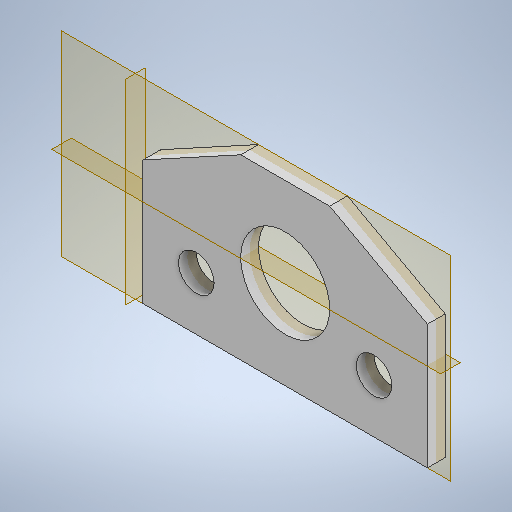
# Autodesk Inventor part: chap2ex3
Saved by Autodesk Inventor 2025.2 (Build 292293000, 293)
## iProperties
Created: 2025-01-31
Part Number: chap2ex3
Material: Generic
Document SubType Name: Modeling
Designer: Moofin
Density: 1 g/cm^3
Appearance: Default
Author: Moofin
Autodesk Inventor part; units mm, degrees
sketch "Sketch1" plane through (0, 0, 0) normal (0, 0, 1) x (1, 0, 0)
  line L0 (5.8796, 31.75) -> (107.4796, 31.75)
  line L1 (107.4796, 31.75) -> (107.4796, -31.75)
  line L2 (107.4796, -31.75) -> (5.8796, -31.75)
  line L3 (5.8796, -31.75) -> (5.8796, 31.75)
  line L4 (-21.4959, 0) -> (128.9756, 0) projected
  point P0 (0, 0)
  dimension "d0" = 63.5
  dimension "d1" = 101.6
  dimension "d2" = 31.75
  constraints: 8 end point, 2 parallel, 1 horizontal, 1 perpendicular
  measures "d0" distance between parallel lines of L2 L0
  measures "d1" distance between parallel lines of L1 L3
  measures "d2" distance between parallel lines of L4 L0
extrude "Extrusion1" add sketch "Sketch1" along normal mid plane 6.35
sketch "Sketch2" plane through (0, 0, 3.175) normal (0, 0, 1) x (1, 0, 0)
  circle A0 centre (56.6796, 0) radius 15.875
  circle A1 centre (24.9296, -12.7) radius 6.35
  line L0 (5.8796, -31.75) -> (107.4796, -31.75) projected
  line L1 (5.8796, 31.75) -> (5.8796, -31.75) projected
  circle A2 centre (88.4296, -12.7) radius 6.35
  line L2 (107.4796, -31.75) -> (107.4796, 31.75) projected
  line L3 (107.4796, 31.75) -> (5.8796, 31.75) projected
  point P0 (0, 0)
  dimension "d5" = 31.75
  dimension "d6" = 12.7
  dimension "d8" = 19.05
  dimension "d9" = 19.05
  dimension "d10" = 12.7
  dimension "d11" = 19.05
  dimension "d12" = 19.05
  dimension "d13" = 31.75
  dimension "d14" = 50.8
  constraints: 3 centre point
  measures "d5" diameter of A0
  measures "d6" diameter of A1
  measures "d8" distance from line of L0 A1.centre
  measures "d9" distance from line of A1.centre L1
  measures "d10" diameter of A2
  measures "d11" distance from line of L2 A2.centre
  measures "d12" distance from line of A2.centre L0
  measures "d13" distance from line of L3 A0.centre
  measures "d14" distance from line of L2 A0.centre
extrude "Extrusion2" cut sketch "Sketch2" against normal up to surface (6.35 mm away) contours A0 | A1 | A2
chamfer "Chamfer1" distance 19.05 distance2 34.925 1 edges at (107.4796, 31.75, 0) measured on face at (107.4796, 10.5833, 1.0583)
chamfer "Chamfer2" distance 34.925 distance2 19.05 1 edges at (5.8796, 31.75, 0) measured on face at (50.3296, 31.75, 1.0583)
equation "\"d2\" = 0.5 * d0"
equation "\"d9\" = d8"
equation "\"d11\" = d8"
equation "\"d12\" = d8"
body "Solid1"
